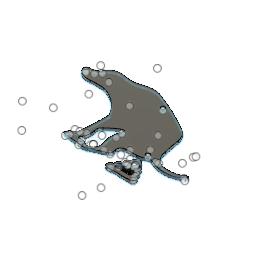
Dog and Poo (Autodesk Fusion 360 design; units mm, degrees)
Autodesk Fusion 360 part; units mm, degrees
sketch "Sketch1" plane through (0, 0, 0) normal (0, 0, 1) x (1, 0, 0)
  arc A0 (-134, 66.3961) -> (-144.4757, 66.3961) centre (-139.2379, 8.441) ccw
  arc A1 (-114.2616, 50.7799) -> (-134, 66.3961) centre (-142.2278, 35.714) ccw
  line L0 (-114.2616, 50.7799) -> (-114.0288, 49.7229)
  arc A2 (-115, 28) -> (-114.0288, 49.7229) centre (-275.457, 46.0573) ccw
  arc A3 (-118.5, 25) -> (-115, 28) centre (-119.3632, 29.5487) ccw
  arc A4 (-118.5, 25) -> (-119.1324, 24.1529) centre (-118.1854, 24.1055) ccw
  line L1 (-119.1324, 24.1529) -> (-120, 22)
  arc A5 (-120, 22) -> (-119.5, 21) centre (-119.1183, 21.8159) ccw
  line L2 (-119.5, 21) -> (-104.5821, 19.4083)
  arc A6 (-104.5821, 19.4083) -> (-100, 20) centre (-103.0136, 25.3002) ccw
  arc A7 (-89, 25) -> (-100, 20) centre (465.9698, -1210.5336) ccw
  arc A8 (-89, 25) -> (-87.7072, 27.2196) centre (-89.4311, 26.7374) ccw
  arc A9 (-87.7072, 27.2196) -> (-88.2972, 29.8156) centre (-94.4337, 27.0559) ccw
  arc A10 (-85, 34) -> (-88.2972, 29.8156) centre (-84.7438, 30.4069) ccw
  arc A11 (-85, 34) -> (-76.6139, 34.2209) centre (-103.445, 893.5026) ccw
  arc A12 (-76.6139, 34.2209) -> (-70, 36.5) centre (-76.6214, 44.9788) ccw
  arc A13 (-70, 36.5) -> (-66.9885, 36.5693) centre (-87.0109, 841.1339) ccw
  arc A14 (-66.9885, 36.5693) -> (-42.1124, 37.486) centre (-55.2736, 56.6498) ccw
  arc A15 (-42.1124, 37.486) -> (-41.9352, 39.7017) centre (-44.6763, 38.8061) ccw
  arc A16 (-41.9352, 39.7017) -> (-44.5645, 38.8745) centre (-42.7162, 37.5921) ccw
  arc A17 (-59.5, 37) -> (-44.5645, 38.8745) centre (-54.5602, 58.0793) ccw
  arc A18 (-67.5, 47.5) -> (-59.5, 37) centre (-55.3956, 48.4248) ccw
  arc A19 (-70, 60) -> (-67.5, 47.5) centre (32.5, 74) ccw
  arc A20 (-70, 60) -> (-77.9596, 69.8396) centre (-83.176, 57.4806) ccw
  arc A21 (-77.9596, 69.8396) -> (-106.3794, 83.2518) centre (-175.3693, -99.7498) ccw
  arc A22 (-106.3794, 83.2518) -> (-121, 83.5) centre (-113.9802, 66.2585) ccw
  arc A23 (-132.5, 82.5) -> (-121, 83.5) centre (-128.4183, 102.1853) ccw
  arc A24 (-132.5, 82.5) -> (-139, 83) centre (-137.6135, 58.5251) ccw
  arc A25 (-139, 83) -> (-146.1929, 77.2529) centre (-137.7525, 74.0638) ccw
  arc A26 (-152.5, 74.5) -> (-146.1929, 77.2529) centre (-152.079, 82.1368) ccw
  arc A27 (-152.5, 74.5) -> (-154.5, 74) centre (-152.7867, 71.397) ccw
  arc A28 (-154.5, 74) -> (-155.5, 72) centre (-153.9561, 72.478) ccw
  arc A29 (-155.5, 72) -> (-153, 68.5) centre (-148.8874, 74.0804) ccw
  arc A30 (-153, 68.5) -> (-144.4757, 66.3961) centre (-146.23, 77.6091) ccw
  arc A31 (-100.0068, 45.6188) -> (-107.7004, 39.4639) centre (-70.4113, 0.7385) ccw
  arc A32 (-98, 46) -> (-100.0068, 45.6188) centre (-97.8945, 39.9724) ccw
  arc A33 (-97.4056, 44.0068) -> (-98, 46) centre (-98.4612, 44.7772) ccw
  arc A34 (-97.4056, 44.0068) -> (-98.4681, 32.7228) centre (-84.236, 37.0748) ccw
  arc A35 (-98.4681, 32.7228) -> (-97.2591, 28.07) centre (-64.2405, 39.1331) ccw
  arc A36 (-101, 22) -> (-97.2591, 28.07) centre (-102.3157, 26.9986) ccw
  arc A37 (-105.2091, 22.7944) -> (-101, 22) centre (-102.3081, 26.6173) ccw
  arc A38 (-105.2091, 22.7944) -> (-108.7995, 23.6737) centre (-107.6074, 20.7712) ccw
  arc A39 (-110.1184, 23.2707) -> (-108.7995, 23.6737) centre (-111.9116, 31.4993) ccw
  arc A40 (-110.0085, 25.9085) -> (-110.1184, 23.2707) centre (-109.441, 24.5637) ccw
  arc A41 (-110.0085, 25.9085) -> (-108.7995, 31.4406) centre (-116.1933, 30.1583) ccw
  arc A42 (-108.7995, 31.4406) -> (-109.0926, 34.4814) centre (-158.5345, 28.1814) ccw
  arc A43 (-107.7004, 39.4639) -> (-109.0926, 34.4814) centre (-104.988, 36.0203) ccw
  circle A44 centre (-71.5, 27.5) radius 1.5
  circle A45 centre (-72.5, 39) radius 1.5
  arc A46 (-65, 24) -> (-67.5, 27.5) centre (-67.1216, 25.1274) ccw
  arc A47 (-62.5, 20) -> (-65, 24) centre (-64.9893, 21.2255) ccw
  arc A48 (-62.5, 15) -> (-62.5, 20) centre (-62.607, 17.5) ccw
  arc A49 (-67.5, 27.5) -> (-74.5, 33) centre (-74.5238, 25.7652) ccw
  arc A50 (-73.9458, 31.3835) -> (-74.5, 33) centre (-78.1441, 30.8474) ccw
  arc A51 (-73.9458, 31.3835) -> (-75, 28) centre (-72.0902, 28.9494) ccw
  arc A52 (-75, 28) -> (-77.1291, 24.2591) centre (-75.1536, 25.6111) ccw
  arc A53 (-77.1291, 24.2591) -> (-79.9485, 20.0147) centre (-76.9676, 21.0932) ccw
  arc A54 (-79.9485, 20.0147) -> (-79.9485, 14.8609) centre (-79.9605, 17.4378) ccw
  arc A55 (-79.9485, 14.8609) -> (-76.3408, 14.8306) centre (-78.0448, 26.7383) ccw
  arc A56 (-68.9435, 14.8609) -> (-76.3408, 14.8306) centre (-72.5331, -11.7799) ccw
  arc A57 (-68.9435, 14.8609) -> (-62.5, 15) centre (-66.2313, 38.5289) ccw
  circle A58 centre (-98, 76) radius 1.5
  dimension "d1" = 3
  dimension "d2" = 3
  dimension "d3" = 3
  constraint tangent A11 A13
  constraint tangent A14 A17
  constraint tangent A20 A22
  constraint tangent A31 A34
  constraint tangent A55 A56
  measures "d1" diameter of A44
  measures "d2" diameter of A45
  measures "d3" diameter of A58
extrude "Extrude1" add sketch "Sketch1" along normal blind 2 contours A0 A1 L0 A2 A3 A4 L1 A5 L2 A6 A7 A8 A9 A10 A11 A12 A13 A14 A15 A16 A17 A18 A19 A20 A21 A22 A23 A24 A25 A26 A27 A28 A29 A30 makes body 1
extrude "Extrude2" add sketch "Sketch1" along normal blind 2 separate body contours A46 A47 A48 A49 A50 A51 A52 A53 A54 A55 A56 A57 makes body 2
ref_plane "WorkPlane1" through (-71.5217, 23.7453, 12) normal (0, 0, 1) x (1, 0, 0)
sketch "Sketch3" plane through (0, 0, 2) normal (0, 0, 1) x (-1, 0, 0)
  circle A0 centre (71.5, -27.5) radius 1.5
  arc A1 (73.9458, -31.3835) -> (75, -28) centre (72.0902, -28.9494) ccw
  arc A2 (75, -28) -> (77.1291, -24.2591) centre (75.1536, -25.6111) ccw
  arc A3 (77.1291, -24.2591) -> (79.9485, -20.0147) centre (76.9676, -21.0932) ccw
  arc A4 (79.9485, -20.0147) -> (79.9485, -14.8609) centre (79.9605, -17.4378) ccw
  arc A5 (79.9485, -14.8609) -> (76.3408, -14.8306) centre (78.0448, -26.7383) ccw
  arc A6 (68.9435, -14.8609) -> (76.3408, -14.8306) centre (72.5331, 11.7799) ccw
  arc A7 (68.9435, -14.8609) -> (62.5, -15) centre (66.2313, -38.5289) ccw
  arc A8 (62.5, -15) -> (62.5, -20) centre (62.607, -17.5) ccw
  arc A9 (62.5, -20) -> (65, -24) centre (64.9893, -21.2255) ccw
  arc A10 (65, -24) -> (67.5, -27.5) centre (67.1216, -25.1274) ccw
  arc A11 (67.5, -27.5) -> (74.5, -33) centre (74.5238, -25.7652) ccw
  arc A12 (73.9458, -31.3835) -> (74.5, -33) centre (78.1441, -30.8474) ccw
  line L0 (77.2341, -17) -> (65, -17) construction
  line L1 (65, -17) -> (65, -22.1925) construction
  line L2 (65, -22.1925) -> (77.2341, -22.1925) construction
  line L3 (77.2341, -22.1925) -> (77.2341, -17) construction
  text T0 "2020" font "Arial" height 4 align left top in box 12.2341 x 5.1925 at (77.2341, -17) x (-1, 0) y (0, -1) spacing 1
emboss "Emboss1" depth 0.5 profiles "Sketch3" section 1 text T0 onto face at (-68.3699, 21.6328, 2) on bodies 2 bodies 2
